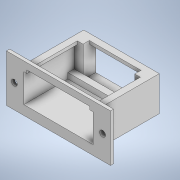
# Autodesk Inventor part: External interface bottom
Saved by Autodesk Inventor 2020 (Build 240168000, 168)
## iProperties
Created: 2019-06-27
Part Number: External interface bottom
Material: Generic
Document SubType Name: Modeling
Designer: cruss
Density: 1 g/cm^3
Appearance: Default
Author: cruss
## iProperties of the stored document _3DPrint.ipt
Created: 2019-07-11
Part Number: _3DPrint
Material: Generic
Document SubType Name: Modeling
Designer: cruss
Density: 1 g/cm^3
Appearance: Default
Author: cruss
Autodesk Inventor part; units mm, degrees
ref_plane "YZ Plane" through (0, 0, 0) normal (1, 0, 0) x (0, 1, 0)
ref_plane "XZ Plane" through (0, 0, 0) normal (0, 1, 0) x (-1, 0, 0)
ref_plane "XY Plane" through (0, 0, 0) normal (0, 0, 1) x (1, 0, 0)
sketch "Sketch1" plane through (0, 0, 0) normal (0, 0, 1) x (1, 0, 0)
  line L0 (0, 0) -> (-41.91, 0)
  line L1 (-41.91, 0) -> (-41.91, 19.05)
  line L2 (-41.91, 19.05) -> (0, 19.05)
  line L3 (0, 19.05) -> (0, 0)
  circle A0 centre (-38.735, 9.525) radius 1.1938
  circle A1 centre (-3.175, 9.525) radius 1.1938
  dimension "d0" = 41.91
  dimension "d1" = 19.05
  dimension "d2" = 2.3876
  dimension "d3" = 2.3876
  dimension "d4" = 3.175
  dimension "d5" = 3.175
  dimension "d6" = 9.525
  dimension "d7" = 9.525
  constraints: 8 end point, 2 centre point, 2 parallel, 1 horizontal, 1 perpendicular
  measures "d0" distance of L1.end L2.end
  measures "d1" distance of L0.end L1.end
  measures "d2" diameter of A0
  measures "d3" diameter of A1
  measures "d4" distance from line of L1 A0.centre
  measures "d5" distance from line of L3 A1.centre
  measures "d6" distance from line of L2 A0.centre
  measures "d7" distance from line of L2 A1.centre
extrude "Extrusion1" add sketch "Sketch1" against normal blind 1.27
sketch "Sketch2" plane through (0, 0, 0) normal (0, 0, 1) x (1, 0, 0)
  line L0 (-41.91, 19.05) -> (-41.91, 0) projected
  line L1 (-36.195, 16.51) -> (-5.715, 16.51)
  line L2 (-5.715, 16.51) -> (-5.715, 2.54)
  line L3 (-5.715, 2.54) -> (-36.195, 2.54)
  line L4 (-36.195, 2.54) -> (-36.195, 16.51)
  line L5 (-41.91, 0) -> (0, 0) projected
  line L6 (0, 0) -> (0, 19.05) projected
  dimension "d31" = 13.97
  dimension "d32" = 2.54
  dimension "d33" = 30.48
  dimension "d34" = 5.715
  constraints: 8 end point, 2 parallel, 1 horizontal, 1 perpendicular
  measures "d31" distance of L3.end L1.start
  measures "d32" distance between parallel lines of L5 L3
  measures "d33" distance of L1.start L1.end
  measures "d34" distance between parallel lines of L6 L2
extrude "Extrusion2" add sketch "Sketch2" against normal blind 25.4
sketch "Sketch3" plane through (0, 0, -25.4) normal (0, 0, -1) x (-1, 0, 0)
  line L0 (6.985, 15.24) -> (34.925, 15.24)
  line L1 (34.925, 15.24) -> (34.925, 3.81)
  line L2 (34.925, 3.81) -> (6.985, 3.81)
  line L3 (6.985, 3.81) -> (6.985, 15.24)
  line L4 (5.715, 16.51) -> (5.715, 2.54) projected
  line L5 (36.195, 16.51) -> (5.715, 16.51) projected
  line L6 (36.195, 2.54) -> (36.195, 16.51) projected
  line L7 (5.715, 2.54) -> (36.195, 2.54) projected
  point P0 (0, 0)
  dimension "d35" = 1.27
  dimension "d36" = 1.27
  dimension "d37" = 1.27
  dimension "d38" = 1.27
  constraints: 8 end point, 2 parallel, 1 horizontal, 1 perpendicular
  measures "d35" distance between parallel lines of L3 L4
  measures "d36" distance between parallel lines of L5 L0
  measures "d37" distance between parallel lines of L6 L1
  measures "d38" distance between parallel lines of L7 L2
extrude "Extrusion3" cut sketch "Sketch3" against normal blind 25.4 contours L0 L1 L2 L3
sketch "Sketch4" plane through (0, 0, 0) normal (0, 0, 1) x (1, 0, 0)
  line L0 (-34.925, 15.24) -> (-6.985, 15.24) projected
  line L1 (-36.195, 16.51) -> (-5.715, 16.51) projected
  line L2 (-33.655, 15.24) -> (-8.255, 15.24)
  line L3 (-8.255, 15.24) -> (-8.255, 16.51)
  line L4 (-8.255, 16.51) -> (-33.655, 16.51)
  line L5 (-33.655, 16.51) -> (-33.655, 15.24)
  line L6 (-34.925, 3.81) -> (-34.925, 15.24) projected
  line L7 (-6.985, 15.24) -> (-6.985, 3.81) projected
  dimension "d39" = 1.27
  dimension "d40" = 1.27
  constraints: 8 end point, 2 parallel, 2 point on line, 1 horizontal, 1 perpendicular
  measures "d39" distance between parallel lines of L6 L5
  measures "d40" distance between parallel lines of L3 L7
extrude "Extrusion4" cut sketch "Sketch4" against normal blind 22.86
sketch "Sketch7" plane through (-34.925, 3.81, -25.4) normal (0, 1, 0) x (1, 0, 0)
  line L0 (0, 0) -> (0, -25.4) projected
  line L1 (26.67, -5.08) -> (0, -5.08)
  line L2 (0, -5.08) -> (0, -7.62)
  line L3 (0, -7.62) -> (26.67, -7.62)
  line L4 (26.67, -7.62) -> (26.67, -5.08)
  line L5 (0, 0) -> (27.94, 0) projected
  line L6 (26.67, -2.54) -> (26.67, -24.13) projected
  point P0 (34.925, -25.4)
  point P1 (0, -5.08)
  dimension "d54" = 2.54
  dimension "d55" = 5.08
  constraints: 8 end point, 2 parallel, 1 horizontal, 1 perpendicular, 1 point on line
  measures "d54" distance between parallel lines of L3 L1
  measures "d55" distance between parallel lines of L5 L1
extrude "Extrusion6" add sketch "Sketch7" along normal blind 2.286
sketch "Sketch8" plane through (-34.925, 3.81, -25.4) normal (0, 1, 0) x (1, 0, 0)
  line L0 (28.0721, -5.08) -> (24.384, -5.08)
  line L1 (24.384, -5.08) -> (24.384, 0)
  line L2 (24.384, 0) -> (27.94, 0)
  line L3 (0, -5.08) -> (3.556, -5.08)
  line L4 (3.556, -5.08) -> (3.556, 0)
  line L5 (3.556, 0) -> (0, 0)
  line L6 (0, 0) -> (0, -5.08)
  line L7 (0, 0) -> (27.94, 0) projected
  line L8 (27.94, 0) -> (27.94, -25.4) projected
  line L9 (27.94, -5.08) -> (27.94, 0)
  point P0 (34.925, -25.4)
  dimension "d46" = 3.556
  dimension "d47" = 5.08
  dimension "d48" = 3.556
  dimension "d49" = 5.08
  constraints: 16 end point, 3 parallel, 2 horizontal, 2 perpendicular, 2 point on line, 1 collinear
  measures "d46" distance of L1.end L2.end
  measures "d47" distance of L0.end L1.end
  measures "d48" distance of L5.end L4.end
  measures "d49" distance of L4.end L3.end
extrude "Extrusion7" add sketch "Sketch8" along normal blind 12.7
sketch "Sketch9" plane through (-31.369, 3.81, -25.4) normal (0, 1, 0) x (1, 0, 0)
  line L0 (0, -5.08) -> (23.114, -5.08) projected
  line L1 (0, 0) -> (20.828, 0) projected
  line L2 (20.828, -5.08) -> (20.828, 0)
  line L3 (20.828, 0) -> (0, 0)
  line L4 (0, 0) -> (0, -5.08)
  line L5 (20.828, -5.08) -> (20.828, 0) projected
  line L6 (0, 0) -> (0, -5.08) projected
  line L7 (20.828, -5.08) -> (0, -5.08)
  point P0 (31.369, -25.4)
  point P1 (20.828, -5.08)
  point P2 (-3.556, 0)
  point P3 (-3.556, -5.08)
  point P4 (24.384, 0)
  constraints: 8 end point, 1 parallel, 1 perpendicular
extrude "Extrusion8" add sketch "Sketch9" along normal blind 0.254
equation "\"d3\" = d2"
equation "\"d5\" = d4"
equation "\"d6\" = 0.5 * d1"
equation "\"d7\" = d6"
equation "\"d36\" = d35"
equation "\"d37\" = d35"
equation "\"d38\" = d36"
equation "\"d49\" = d47"
body "Solid1"
